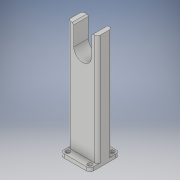
# Autodesk Inventor part: suport lateral
Saved by Autodesk Inventor 2019 (Build 230136000, 136)
## iProperties
Created: 2018-08-16
Part Number: suport lateral
Material: Genérico
Document SubType Name: Modeling
Designer: Albert Garangou Culebras
Density: 1 g/cm^3
Appearance: Valor por defecto
Author: Albert Garangou Culebras
Autodesk Inventor part; units mm, degrees
ref_plane "YZ Plane" through (0, 0, 0) normal (1, 0, 0) x (0, 1, 0)
ref_plane "XZ Plane" through (0, 0, 0) normal (0, 1, 0) x (-1, 0, 0)
ref_plane "XY Plane" through (0, 0, 0) normal (0, 0, 1) x (1, 0, 0)
sketch "Boceto1" plane through (0, 0, 0) normal (0, 1, 0) x (-1, 0, 0)
  line L0 (0, 0) -> (0, -40)
  line L1 (0, -40) -> (-40, -40)
  line L2 (-40, -40) -> (-40, 0)
  line L3 (-40, 0) -> (0, 0)
  dimension "d0" = 40
  dimension "d1" = 40
  dimension "d2" = 40
  constraints: 8 end point, 2 perpendicular, 1 vertical
  measures "d0" distance of L0.start L0.end
  measures "d1" distance of L0.end L1.end
  measures "d2" distance of L1.end L2.end
extrude "Extrusión1" add sketch "Boceto1" along normal blind 5
fillet "Empalme1" radius 5 4 edges at (40, 2.5, 0) (0, 2.5, 0) (40, 2.5, -40) (0, 2.5, -40) curvature continuous yes
sketch "Boceto2" plane through (0, 5, 0) normal (0, 1, 0) x (1, 0, 0)
  line L0 (0, 5) -> (0, 35)
  line L1 (0, 35) -> (0, 5) projected
  line L2 (40, 5) -> (40, 35) projected
  line L3 (40, 4) -> (40, 35)
  line L4 (40, 5) -> (36, 5)
  line L5 (40, 5) -> (35, 5)
  circle A0 centre (35, 5) radius 1.6
  line L6 (0, 5) -> (5, 5)
  line L7 (0, 35) -> (5, 35)
  line L8 (40, 35) -> (35, 35)
  circle A1 centre (5, 5) radius 1.6
  circle A2 centre (5, 35) radius 1.6
  circle A3 centre (35, 35) radius 1.6
  point P0 (0, 0)
  dimension "d6" = 5
  dimension "d7" = 3.2
  dimension "d8" = 5
  dimension "d9" = 5
  dimension "d10" = 5
  dimension "d11" = 3.2
  dimension "d12" = 3.2
  dimension "d13" = 3.2
  constraints: 14 end point, 4 centre point, 4 coincident, 3 horizontal, 1 collinear, 1 perpendicular, 1 point on line, 1 vertical
  measures "d6" distance of L2.start L5.end
  measures "d7" diameter of A0
  measures "d8" distance of L0.start L6.end
  measures "d9" distance of L0.end L7.end
  measures "d10" distance of L2.end L8.end
  measures "d11" diameter of A1
  measures "d12" diameter of A2
  measures "d13" diameter of A3
extrude "Extrusión2" cut sketch "Boceto2" against normal blind 5
sketch "Boceto3" plane through (0, 5, 0) normal (0, 1, 0) x (1, 0, 0)
  circle A0 centre (5, 5) radius 3
  circle A1 centre (5, 35) radius 3
  circle A2 centre (35, 35) radius 3
  circle A3 centre (35, 5) radius 3
  point P0 (0, 0)
  dimension "d16" = 6
  dimension "d17" = 6
  dimension "d18" = 6
  dimension "d19" = 6
  constraints: 4 centre point
  measures "d16" diameter of A0
  measures "d17" diameter of A1
  measures "d18" diameter of A2
  measures "d19" diameter of A3
extrude "Extrusión3" cut sketch "Boceto3" against normal blind 3
sketch "Boceto4" plane through (0, 5, 0) normal (0, 1, 0) x (1, 0, 0)
  line L0 (0, 5) -> (0, 35) projected
  line L1 (0, 20) -> (0, 10)
  line L2 (0, 10) -> (40, 10)
  line L3 (40, 5) -> (40, 35) projected
  line L4 (0, 30) -> (40, 30)
  line L5 (0, 10) -> (0, 30)
  line L6 (40, 10) -> (40, 30)
  point P0 (0, 0)
  constraints: 10 end point, 4 point on line, 2 collinear, 2 perpendicular, 1 midpoint
extrude "Extrusión4" add sketch "Boceto4" along normal blind 150
sketch "Boceto6" plane through (0, 5, -10) normal (0, 0, 1) x (1, 0, 0)
  line L0 (0, 150) -> (40, 150) projected
  line L1 (0, 150) -> (40, 150)
  line L2 (20, 150) -> (10, 150)
  line L3 (20, 150) -> (30, 150)
  line L4 (0, 0) -> (40, 0) projected
  line L5 (10, 110) -> (30, 110)
  line L6 (10, 110) -> (8, 110)
  line L7 (30, 110) -> (32, 110)
  line L8 (32, 110) -> (32, 150)
  line L9 (8, 110) -> (8, 150)
  line L10 (40, 150) -> (0, 150) projected
  point P0 (0, -5)
  dimension "d34" = 20
  dimension "d35" = 2
  dimension "d36" = 2
  constraints: 16 end point, 4 point on line, 2 horizontal, 2 perpendicular, 1 collinear, 1 midpoint
  measures "d34" distance of L5.start L5.end
  measures "d35" distance of L5.start L6.end
  measures "d36" distance of L5.end L7.end
extrude "Extrusión5" cut sketch "Boceto6" against normal blind 150
sketch "Boceto7" plane through (40, 5, -30) normal (0, 0, -1) x (-1, 0, 0)
  line L0 (8, 110) -> (32, 110) projected
  line L1 (10, 120) -> (10, 110)
  line L2 (10, 110) -> (20, 110)
  line L3 (30, 110) -> (20, 110)
  line L4 (32, 110) -> (8, 110) projected
  line L5 (20, 110) -> (20, 122)
  circle A0 centre (20, 122) radius 12
  line L6 (30, 110) -> (32, 110)
  line L7 (8, 150) -> (8, 110) projected
  line L8 (8, 122) -> (8, 110)
  line L9 (8, 110) -> (20, 110)
  line L10 (32, 110) -> (32, 122)
  line L11 (32, 110) -> (32, 150) projected
  point P0 (40, -5)
  dimension "d40" = 12
  constraints: 16 end point, 4 collinear, 3 point on circle, 2 perpendicular, 2 point on line, 1 centre point, 1 coincident, 1 midpoint, 1 tangent
  measures "d40" distance of L2.end L5.end
extrude "Extrusión7" add sketch "Boceto7" against normal blind 20 contours L7 A0 L1 L0 | L1 A0 L0 | A0 L10 L0
chamfer "Chaflán2" distance 2 angle 45 2 edges at (8, 155, -20) (32, 155, -20)
fillet "Empalme2" radius 4 4 edges at (0, 80, -10) (40, 80, -10) (40, 80, -30) (0, 80, -30)
